Encoder mockup_v1 (Autodesk Fusion 360 design; units mm, degrees)
Autodesk Fusion 360 part; units mm, degrees
sketch "Sketch1" plane through (0, 0, 0) normal (0, 0, 1) x (1, 0, 0) in component "Encoder"
  circle A0 centre (0, 0) radius 12
  dimension "d1" = 24
  constraint coincident A0.centre origin
  measures "d1" diameter of A0
extrude "Extrude1" add sketch "Sketch1" along normal blind 24 in component "Encoder"
sketch "Sketch2" plane through (0, 0, 24) normal (0, 0, 1) x (-1, 0, 0) in component "Encoder"
  circle A0 centre (0, 0) radius 12
  circle A1 centre (0, 0) radius 6
  circle A2 centre (0, 0) radius 2
  circle A3 centre (0, 0) radius 9 construction
  line L0 (0, 0) -> (0, 12) construction
  circle A4 centre (0, 9) radius 1.5
  circle A5 centre (-7.7942, -4.5) radius 1.5
  circle A6 centre (7.7942, -4.5) radius 1.5
  dimension "d4" = 12
  dimension "d5" = 4
  dimension "d6" = 18
  dimension "d7" = 3
  dimension "d9" = 360
  constraint concentric A0 A1
  constraint concentric A1 A2
  constraint concentric A1 A3
  constraint coincident A0.centre A1.centre
  constraint coincident A0 L0.end
  constraint vertical L0
  constraint coincident A3 A4.centre
  constraint coincident L0 A4.centre
  measures "d4" diameter of A1
  measures "d5" diameter of A2
  measures "d6" diameter of A3
  measures "d7" diameter of A4
extrude "Extrude2" add sketch "Sketch2" along normal blind 1 contours A1 in component "Encoder"
extrude "Extrude3" cut sketch "Sketch2" against normal blind 6 contours A4 | A5 | A6 in component "Encoder"
extrude "Extrude4" add sketch "Sketch2" along normal blind 10 contours A2 in component "Encoder"
sketch "Sketch3" plane through (0, 0, 0) normal (0, 1, 0) x (1, 0, 0) in component "Encoder"
  line L0 (-12, -24) -> (12, -24)
  line L1 (-12, 0) -> (12, 0)
  line L2 (12, -24) -> (12, -23)
  line L3 (12, -23) -> (11, -23)
  line L4 (11, -23) -> (11, -21.8)
  line L5 (11, -21.8) -> (12, -21.8)
  line L6 (12, -21.8) -> (12, -23)
  dimension "d16" = 1
  dimension "d17" = 1
  dimension "d18" = 1.2
  constraint coincident L0.end L2.start
  constraint perpendicular L0 L2
  constraint perpendicular L2 L3
  constraint perpendicular L3 L4
  constraint perpendicular L2 L5
  constraint perpendicular L3 L6
  measures "d16" distance of L0.end L2.end
  measures "d17" distance of L2.end L3.end
  measures "d18" distance of L3.end L4.end
revolve "Revolve1" cut sketch "Sketch3" angle 360 about axis through (0, 0, 0) along (0, 0, -1) in component "Encoder"
component "Encoder" placed x (1, 0, 0) y (0, 1, 0) z (0, 0, 1) at (0, 0, 0)
equation "d14 = 1 mm + 9 mm"
